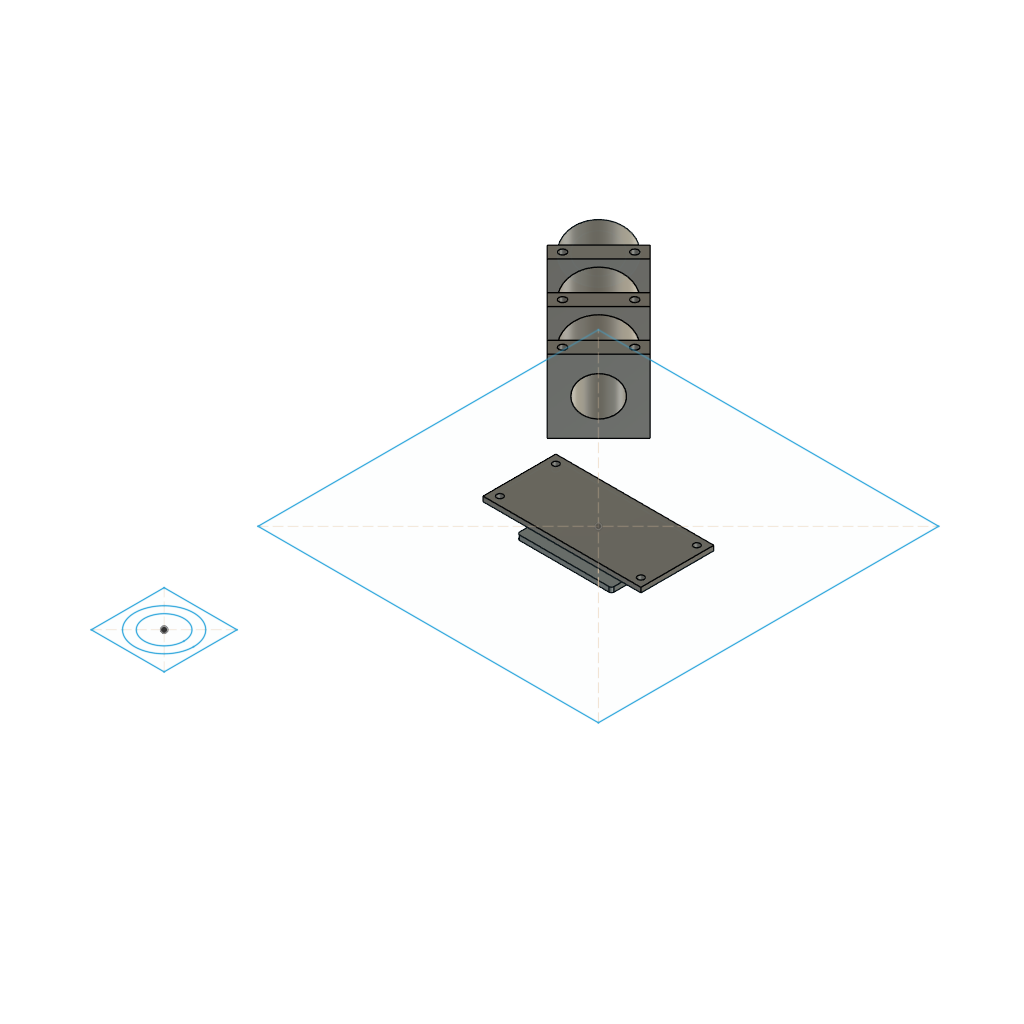
Katlanma Mekanizması (Autodesk Fusion 360 design; units mm, degrees)
Autodesk Fusion 360 part; units mm, degrees
note: some values were not read from the file. Set by a fixed rule: which sketch regions a step uses.
sketch "Sketch1" plane through (0, 0, 0) normal (0, 0, 1) x (1, 0, 0)
  line L0 (48.1033, 9.878) -> (11.2527, 9.878)
  line L1 (11.2527, 42.4871) -> (48.1033, 42.4871)
  line L2 (49.1355, 41.4549) -> (49.1355, 10.9102)
  line L3 (8.569, 19.0428) -> (8.0309, 19.0428)
  line L4 (5.76, 21.3137) -> (5.76, 30.6887)
  line L5 (8.0309, 32.9595) -> (8.569, 32.9595)
  line L6 (10.2205, 10.9102) -> (10.2205, 17.3913)
  line L7 (10.2205, 34.611) -> (10.2205, 41.4549)
  arc A0 (8.569, 32.9595) -> (10.2205, 34.611) centre (8.569, 34.611) ccw
  arc A1 (10.2205, 17.3913) -> (8.569, 19.0428) centre (8.569, 17.3913) ccw
  arc A2 (11.2527, 42.4871) -> (10.2205, 41.4549) centre (11.2527, 41.4549) ccw
  arc A3 (49.1355, 41.4549) -> (48.1033, 42.4871) centre (48.1033, 41.4549) ccw
  arc A4 (48.1033, 9.878) -> (49.1355, 10.9102) centre (48.1033, 10.9102) ccw
  arc A5 (10.2205, 10.9102) -> (11.2527, 9.878) centre (11.2527, 10.9102) ccw
  arc A6 (8.0309, 32.9595) -> (5.76, 30.6887) centre (8.0309, 30.6887) ccw
  arc A7 (5.76, 21.3137) -> (8.0309, 19.0428) centre (8.0309, 21.3137) ccw
  circle A8 centre (19.7019, 36.2604) radius 2
  circle A9 centre (39.7001, 36.2604) radius 2
  circle A10 centre (19.7019, 16.2604) radius 2
  circle A11 centre (39.7001, 16.2604) radius 2
  dimension "d5" = 4
  dimension "d6" = 4
  dimension "d7" = 4
  dimension "d8" = 4
  constraint horizontal L0
  constraint vertical L6
  constraint horizontal L1
  constraint vertical L2
  constraint horizontal L3
  constraint vertical L4
  constraint horizontal L5
  constraint collinear L6 L7
  constraint tangent L5 A0
  constraint tangent L7 A0
  constraint tangent L3 A1
  constraint tangent L6 A1
  constraint equal A0 A1
  constraint tangent L1 A2
  constraint tangent L7 A2
  constraint tangent L1 A3
  constraint tangent L2 A3
  constraint equal A2 A3
  constraint tangent L0 A4
  constraint tangent L2 A4
  constraint equal A2 A4
  constraint tangent L0 A5
  constraint tangent L6 A5
  constraint equal A2 A5
  constraint tangent L4 A6
  constraint tangent L5 A6
  constraint tangent L3 A7
  constraint tangent L4 A7
  constraint equal A6 A7
  measures "d5" diameter of A8
  measures "d6" diameter of A9
  measures "d7" diameter of A10
  measures "d8" diameter of A11
extrude "Extrude1" add sketch "Sketch1" along normal blind 2 makes body 1
sketch "Sketch2" plane through (0, 0, 0) normal (0, 0, 1) x (1, 0, 0)
  line L0 (75, 0) -> (105, 0)
  line L1 (105, 0) -> (105, 65)
  line L2 (105, 65) -> (75, 65)
  line L3 (75, 65) -> (75, 0)
  line L4 (75, 0) -> (78.5, 0)
  line L5 (75, 3.5) -> (75, 0)
  circle A0 centre (78.5, 3.5) radius 1.3
  line L6 (105, 0) -> (101.5, 0)
  line L7 (105, 3.5) -> (105, 0)
  circle A1 centre (101.5, 3.5) radius 1.3
  line L8 (75, 65) -> (78.5, 65)
  line L9 (75, 61.5) -> (75, 65)
  line L10 (105, 65) -> (101.5, 65)
  line L11 (105, 61.5) -> (105, 65)
  circle A2 centre (78.5, 61.5) radius 1.3
  circle A3 centre (101.5, 61.5) radius 1.3
  dimension "d11" = 30
  dimension "d12" = 65
  dimension "d14" = 3.5
  dimension "d15" = 3.5
  dimension "d16" = 2.6
  dimension "d17" = 3.5
  dimension "d18" = 3.5
  dimension "d19" = 2.6
  dimension "d20" = 3.5
  dimension "d21" = 3.5
  dimension "d22" = 3.5
  dimension "d23" = 3.5
  dimension "d24" = 2.6
  dimension "d25" = 2.6
  constraint horizontal L0
  constraint vertical L1
  constraint horizontal L2
  constraint vertical L3
  constraint horizontal L4
  constraint vertical L5
  constraint horizontal L6
  constraint vertical L7
  constraint horizontal L8
  constraint vertical L9
  constraint horizontal L10
  constraint vertical L11
  measures "d11" distance of L0.start L0.end
  measures "d12" distance of L0.start L2.end
  measures "d14" distance of L0.start L4.end
  measures "d15" distance of L0.start L5.start
  measures "d16" diameter of A0
  measures "d17" distance of L0.end L6.end
  measures "d18" distance of L0.end L7.start
  measures "d19" diameter of A1
  measures "d20" distance of L2.end L8.end
  measures "d21" distance of L2.end L9.start
  measures "d22" distance of L1.end L10.end
  measures "d23" distance of L1.end L11.start
  measures "d24" diameter of A2
  measures "d25" diameter of A3
extrude "Extrude2" add sketch "Sketch2" along normal blind 2 separate body makes body 2
sketch "Sketch3" plane through (0, 0, 2) normal (0, 0, 1) x (-1, 0, 0)
  circle A0 centre (-78.5, -3.5) radius 1.3
  circle A1 centre (-78.5, -61.5) radius 1.3
  circle A2 centre (-101.5, -61.5) radius 1.3
  circle A3 centre (-101.5, -3.5) radius 1.3
  line L0 (-105, 0) -> (-105, -65)
  line L1 (-105, -65) -> (-75, -65)
  line L2 (-75, -65) -> (-75, 0)
  line L3 (-75, 0) -> (-105, 0)
  circle A4 centre (-78.5, -3.5) radius 2.5
  dimension "d28" = 5
  constraint concentric A0 A4
  measures "d28" diameter of A4
move_body "Move1" bodies 2 to x (1, 0, 0) y (0, 1, 0) z (0, 0, 1) at (-25, -4, 0)
move_body "Move2" bodies 2 to x (1, 0, 0) y (0, 1, 0) z (0, 0, 1) at (-0.8645, -2.3175, 0)
move_body "Move3" bodies 2 to x (0, 1, 0) y (-1, 0, 0) z (0, 0, 1) at (125.318, -37.953, 0)
move_body "Move4" bodies 2 to x (1, 0, 0) y (0, 1, 0) z (0, 0, 1) at (-71.6877, 0, 0)
move_body "Move5" bodies 2 to x (1, 0, 0) y (0, 1, 0) z (0, 0, 1) at (0, 0, -5)
move_body "Move6" bodies 2 to x (1, 0, 0) y (0, 1, 0) z (0, 0, 1) at (0, 0, 10)
sketch "Sketch4" plane through (0, 0, 5) normal (0, 0, -1) x (1, 0, 0)
  circle A0 centre (56.4478, -14.6825) radius 1.3
  circle A1 centre (-1.5522, -14.6825) radius 1.3
  circle A2 centre (-1.5522, -37.6825) radius 1.3
  circle A3 centre (56.4478, -37.6825) radius 1.3
  line L0 (-5.0522, -41.1825) -> (59.9478, -41.1825)
  line L1 (59.9478, -41.1825) -> (59.9478, -11.1825)
  line L2 (59.9478, -11.1825) -> (-5.0522, -11.1825)
  line L3 (-5.0522, -11.1825) -> (-5.0522, -41.1825)
  line L4 (97.4478, 43.8175) -> (-42.5522, 43.8175)
  line L5 (-42.5522, 43.8175) -> (-42.5522, -96.1825)
  line L6 (-42.5522, -96.1825) -> (97.4478, -96.1825)
  line L7 (97.4478, -96.1825) -> (97.4478, 43.8175)
  line L8 (97.4478, 43.8175) -> (-42.5522, -96.1825) construction
  line L9 (-42.5522, 43.8175) -> (97.4478, -96.1825) construction
  point P0 (27.4478, -26.1825)
  dimension "d29" = 140
  dimension "d30" = 140
  constraint horizontal L4
  constraint perpendicular L4 L5
  constraint parallel L4 L6
  constraint parallel L5 L7
  constraint coincident L8 P0
  constraint coincident L9 P0
  measures "d29" distance of L5.end L6.end
  measures "d30" distance of L4.end L5.end
sketch "Sketch5" plane through (0, 0, 5) normal (0, 0, -1) x (1, 0, 0)
  circle A0 centre (-25, 100) radius 8.1
  circle A1 centre (-25, 100) radius 12.1
  line L0 (-10, 115) -> (-40, 115)
  line L1 (-40, 115) -> (-40, 85)
  line L2 (-40, 85) -> (-10, 85)
  line L3 (-10, 85) -> (-10, 115)
  line L4 (-10, 115) -> (-40, 85) construction
  line L5 (-40, 115) -> (-10, 85) construction
  point P0 (-25, 100)
  dimension "d31" = 16.2
  dimension "d32" = 24.2
  dimension "d33" = 30
  dimension "d34" = 30
  constraint concentric A0 A1
  constraint horizontal L0
  constraint perpendicular L0 L1
  constraint parallel L0 L2
  constraint parallel L1 L3
  constraint coincident L4 P0
  constraint coincident L5 P0
  constraint coincident P0 A0.centre
  measures "d31" diameter of A0
  measures "d32" diameter of A1
  measures "d33" distance of L1.end L2.end
  measures "d34" distance of L0.end L1.end
extrude "Extrude3" add sketch "Sketch5" against normal blind 7 separate body contours A1 | L0 L1 L2 L3 makes body 3
extrude "Extrude4" add sketch "Sketch5" against normal blind 55 separate body contours A1 makes body 4
sketch "Sketch6" plane through (0, -115, 0) normal (0, -1, 0) x (1, 0, 0)
  line L0 (-40, 5) -> (-10, 5)
  line L1 (-10, 5) -> (-10, 12)
  line L2 (-10, 12) -> (-40, 12)
  line L3 (-40, 12) -> (-40, 5)
  line L4 (-40, 8.5) -> (-10, 8.5)
  line L5 (-40, 8.5) -> (-37, 8.5)
  line L6 (-10, 8.5) -> (-13, 8.5)
  circle A0 centre (-35.5, 8.5) radius 1.5
  circle A1 centre (-14.5, 8.5) radius 1.5
  dimension "d39" = 3
  dimension "d40" = 3
  constraint midpoint L3 L4.start
  constraint midpoint L1 L4.end
  constraint coincident L4 L5.end
  constraint coincident L4 L6.end
  constraint coincident L5.end A0
  constraint coincident L6.end A1
  measures "d39" diameter of A0
  measures "d40" diameter of A1
extrude "Extrude5" cut sketch "Sketch6" against normal blind 10 contours L4 A0 | L4 A0 | L4 A1 | L4 A1 bodies 3 4
sketch "Sketch7" plane through (0, -85, 0) normal (0, 1, 0) x (-1, 0, 0)
  line L0 (10, 5) -> (40, 5)
  line L1 (40, 5) -> (40, 12)
  line L2 (40, 12) -> (10, 12)
  line L3 (10, 12) -> (10, 5)
  line L4 (40, 8.5) -> (10, 8.5)
  line L5 (40, 8.5) -> (37, 8.5)
  line L6 (10, 8.5) -> (13, 8.5)
  circle A0 centre (35.5, 8.5) radius 1.5
  circle A1 centre (14.5, 8.5) radius 1.5
  dimension "d43" = 3
  dimension "d44" = 3
  dimension "d45" = 3
  dimension "d46" = 3
  constraint midpoint L1 L4.start
  constraint midpoint L3 L4.end
  constraint perpendicular L1 L5
  constraint perpendicular L3 L6
  constraint coincident L5.end A0
  constraint coincident L6.end A1
  measures "d43" distance of L4.start L5.end
  measures "d44" distance of L4.end L6.end
  measures "d45" diameter of A0
  measures "d46" diameter of A1
extrude "Extrude6" cut sketch "Sketch7" against normal blind 10 contours L4 A1 | L4 A1 | L4 A0 | L4 A0 bodies 3 4
copy_body "CopyPasteBodies1" bodies 3 makes body 5
move_body "Move7" bodies 5 to x (1, 0, 0) y (0, 1, 0) z (0, 0, 1) at (0, 0, 48)
copy_body "CopyPasteBodies2" bodies 3 makes body 6
move_body "Move8" bodies 6 to x (1, 0, 0) y (0, 1, 0) z (0, 0, 1) at (0, 0, 24)
combine "Combine1" operation add target body 5 tool bodies 4
combine "Combine2" operation add target body 6 tool bodies 5
combine "Combine3" operation add target body 3 tool bodies 6
extrude "Extrude7" add sketch "Sketch5" along normal blind 17 contours A1 bodies 3
move_body "Move9" bodies 3 to x (0.707107, 0.707107, 0) y (0, 0, 1) z (0.707107, -0.707107, 0) at (-28.5355, 117.6381, 120)
sketch "Sketch8" plane through (-81.5721, 81.5721, 0) normal (-0.707107, 0.707107, 0) x (-0.707107, -0.707107, 0)
  circle A0 centre (-38.0051, 20) radius 8.1
  circle A1 centre (-38.0051, 20) radius 12.1
